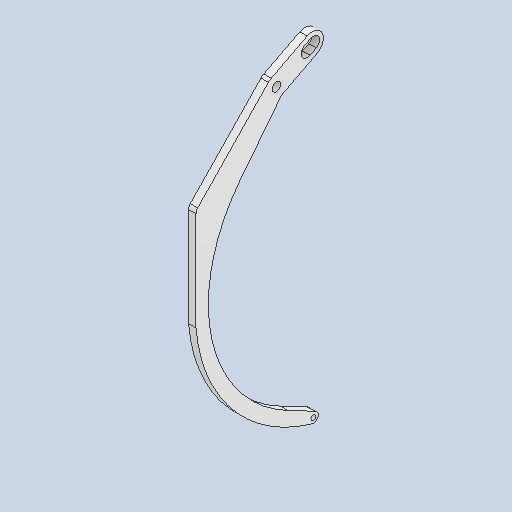
# Autodesk Inventor part: hand-grab-v1-MDF-arm
Saved by Autodesk Inventor 2025.2 (Build 292293000, 293)
## iProperties
Created: 2024-10-30
Part Number: hand-grab-v1-MDF-arm
Material: ABS プラスチック
Document SubType Name: Modeling
Designer: haruy
Density: 1.06 g/cm^3
Appearance: 滑らか - 白
Author: haruy
Autodesk Inventor part; units mm, degrees
ref_plane "YZ Plane" through (0, 0, 0) normal (1, 0, 0) x (0, 1, 0)
ref_plane "XZ Plane" through (0, 0, 0) normal (0, 1, 0) x (-1, 0, 0)
ref_plane "XY Plane" through (0, 0, 0) normal (0, 0, 1) x (1, 0, 0)
derived "hand-grab-v3-Sketch-Base.ipt"
sketch "スケッチ1" plane through (400, 0, 0) normal (1, 0, 0) x (0, 1, 0)
  circle A0 centre (0, 0) radius 120 construction
  circle A1 centre (-96.5237, 35.1318) radius 6.5
  line L0 (0, 0) -> (-96.5237, 35.1318)
  line L1 (0, 0) -> (0, 120)
  line L2 (246.0862, 200) -> (-251.4603, 200)
  circle A2 centre (-67.6203, 200) radius 6.5
  line L3 (0, 0) -> (-120, 0)
  line L4 (248, 9.15) -> (186, 9.15)
  line L5 (186, 9.15) -> (186, -9.15)
  line L6 (186, -9.15) -> (248, -9.15)
  line L7 (248, -9.15) -> (248, 9.15)
  line L8 (186, 5.15) -> (178, 5.15)
  line L9 (178, 5.15) -> (178, -4.85)
  line L10 (178, -4.85) -> (186, -4.85)
  line L11 (186, -4.85) -> (186, 5.15)
  line L12 (178, 3.15) -> (173, 3.15)
  line L13 (173, 3.15) -> (173, -2.85)
  line L14 (173, -2.85) -> (178, -2.85)
  line L15 (178, -2.85) -> (178, 3.15)
  line L16 (173, 2.65) -> (158, 2.65)
  line L17 (158, 2.65) -> (158, -2.35)
  line L18 (158, -2.35) -> (173, -2.35)
  line L19 (173, -2.35) -> (173, 2.65)
  line L20 (186, 34.15) -> (184, 34.15)
  line L21 (184, 34.15) -> (184, -47.85)
  line L22 (184, -47.85) -> (186, -47.85)
  line L23 (186, -47.85) -> (186, 34.15)
  circle A3 centre (150, 65) radius 4 construction
  circle A4 centre (150, 65) radius 14 construction
  line L24 (186, 34.15) -> (191, 34.15)
  line L25 (191, 34.15) -> (191, 14.15)
  line L26 (191, 14.15) -> (186, 14.15)
  line L27 (186, 14.15) -> (186, 34.15)
  line L28 (184, 34.15) -> (147.5804, 61.8148) construction
  line L29 (151.3835, 68.7531) -> (191, 54.15) construction
  line L30 (191, 54.15) -> (191, 34.15)
  line L31 (239.3868, 130) -> (-239.3868, 130)
  circle A5 centre (-96.5237, 35.1318) radius 4
  circle A6 centre (150, 65) radius 9
  line L32 (-92.7649, 33.7637) -> (-100.2825, 36.4998)
  line L33 (165, 36) -> (150, 36) construction
  circle A7 centre (150, 36) radius 5 construction
  circle A8 centre (150, 36) radius 9 construction
  circle A9 centre (-98.8174, 128.095) radius 6.5
  circle A10 centre (165, 36) radius 5 construction
  line L34 (150, 65) -> (165, 36) construction
  circle A11 centre (165, 36) radius 9
  circle A12 centre (150, 65) radius 41.6497 construction
  line L35 (150, 65) -> (150, 36) construction
  line L36 (150, 65) -> (-96.5237, 35.1318) construction
  line L37 (-98.8174, 128.095) -> (150, 65) construction
  line L38 (150, 65) -> (150, 23.3503)
  circle A13 centre (150, 65) radius 32.6497 construction
  circle A14 centre (150, 32.3503) radius 9 construction
  line L39 (166.9362, 23.3503) -> (134.8586, 23.3503)
  line L40 (174, 3.15) -> (174, -2.85)
  circle A15 centre (-96.5237, 35.1318) radius 2
  circle A16 centre (150, 65) radius 3.5
  circle A17 centre (150, 65) radius 29 construction
  circle A18 centre (163.3233, 39.2417) radius 5 construction
  circle A19 centre (162.8638, 40.1299) radius 5
  line L41 (150, 65) -> (169.1348, 28.006) construction
  circle A20 centre (165.4594, 35.1118) radius 5
  line L42 (167.3049, 42.427) -> (169.9005, 37.4089)
  line L43 (158.4228, 37.8328) -> (161.0183, 32.8147)
  circle A21 centre (25, 0) radius 120
  circle A22 centre (25, 0) radius 122.5
  circle A23 centre (25, 0) radius 130.5
  line L44 (-92.7649, 33.7637) -> (-81.3303, 55.6226)
  line L45 (25, 130.5) -> (95, 130.5)
  line L46 (95, 130.5) -> (156.2451, 71.4806)
  line L47 (157.994, 69.1348) -> (172.994, 40.1348)
  line L48 (157.006, 31.8652) -> (142.006, 60.8652)
  line L49 (142.006, 60.8652) -> (98.8819, 94.5593)
  circle A24 centre (123.9097, 89.024) radius 1.5
  circle A25 centre (25, 125.5) radius 1.5
  circle A26 centre (-61, 92) radius 1.5
  line L50 (170, -52.2973) -> (211.3465, -67.3462)
  line L51 (211.3465, -67.3462) -> (205.1901, -84.2607)
  line L52 (205.1901, -84.2607) -> (163.8436, -69.2118)
  line L53 (163.8436, -69.2118) -> (170, -52.2973)
  line L54 (166.9218, -60.7546) -> (0, 0)
  line L55 (172.8191, -53.3234) -> (166.6627, -70.2379)
  line L56 (186, -47.85) -> (172.8191, -53.3234)
  line L57 (182.216, -56.7436) -> (176.0596, -73.6581)
  line L58 (186, -47.85) -> (191, -47.85)
  line L59 (191, -47.85) -> (191, -37.85)
  line L60 (191, -37.85) -> (186, -37.85)
  line L61 (186, -37.85) -> (186, -47.85)
  line L62 (191, -47.85) -> (182.216, -56.7436)
  circle A27 centre (221.5, -275) radius 6
  line L63 (211.5, 20) -> (208.5, 20)
  line L64 (208.5, 20) -> (208.5, -53.7075)
  line L65 (208.5, -53.7075) -> (211.5, -53.7075)
  line L66 (211.5, -53.7075) -> (211.5, 20)
  line L67 (211.5, 20) -> (231.5, 20)
  line L68 (231.5, 20) -> (231.5, -53.7075)
  line L69 (231.5, -53.7075) -> (211.5, -53.7075)
  line L70 (211.5, -53.7075) -> (211.5, 20)
  line L71 (-432.3334, -230) -> (-447.3334, -230)
  line L72 (-447.3334, -230) -> (-447.3334, -860)
  line L73 (-447.3334, -860) -> (-432.3334, -860)
  line L74 (-432.3334, -860) -> (-432.3334, -230)
  line L75 (-432.3334, -250) -> (-432.3334, -230)
  line L76 (343, -291.5) -> (278.5, -291.5)
  line L77 (278.5, -291.5) -> (278.5, -334.5)
  line L78 (278.5, -334.5) -> (343, -334.5)
  line L79 (343, -334.5) -> (343, -291.5)
  line L80 (278.5, -291.5) -> (293.5, -291.5)
  line L81 (293.5, -291.5) -> (293.5, -276.5)
  line L82 (293.5, -276.5) -> (278.5, -276.5)
  line L83 (278.5, -276.5) -> (278.5, -291.5)
  line L84 (211.5, -53.7075) -> (231.5, -53.7075)
  line L85 (231.5, -53.7075) -> (231.5, -305) construction
  line L86 (231.5, -305) -> (211.5, -305)
  line L87 (211.5, -305) -> (211.5, -53.7075) construction
  line L88 (-432.3334, -303) -> (-447.3334, -303)
  line L89 (-432.3334, -303) -> (875.6666, -303)
  line L90 (875.6666, -303) -> (875.6666, -323)
  line L91 (875.6666, -323) -> (-432.3334, -323)
  line L92 (-432.3334, -323) -> (-432.3334, -303)
  line L93 (278.5, -334.5) -> (293.5, -334.5)
  line L94 (293.5, -334.5) -> (293.5, -349.5)
  line L95 (293.5, -349.5) -> (278.5, -349.5)
  line L96 (278.5, -349.5) -> (278.5, -334.5)
  line L97 (278.5, -276.5) -> (263.5, -276.5)
  line L98 (263.5, -276.5) -> (263.5, -359.5)
  line L99 (263.5, -359.5) -> (278.5, -359.5)
  line L100 (278.5, -359.5) -> (278.5, -276.5)
  circle A28 centre (221.5, -275) radius 15
  line L101 (231.5, -275) -> (211.5, -275)
  line L102 (211.5, -275) -> (211.5, -305)
  line L103 (211.5, -305) -> (231.5, -305)
  line L104 (231.5, -305) -> (231.5, -275)
  line L105 (226.5, -266.3397) -> (216.5, -283.6603)
  line L106 (242.4808, -298.6603) -> (252.4808, -281.3397)
  line L107 (216.5, -283.6603) -> (242.4808, -298.6603)
  line L108 (-524.3334, 10.1879) -> (-524.3334, -1075.6286)
  line L109 (278.5, -349.5) -> (263.5, -349.5)
  line L110 (278.5, -276.5) -> (225.8253, -260.6372)
  line L111 (263.5, -349.5) -> (209.9279, -284.544)
  line L112 (278.5, -313) -> (263.5, -313)
  circle A29 centre (271, -291.5) radius 1.6
  circle A30 centre (271, -334.5) radius 1.6
  circle A31 centre (221.5, -275) radius 9.1
  circle A32 centre (221.5, -275) radius 50
  circle A33 centre (239.5, -334.8519) radius 12.5
  line L113 (221.5, -275) -> (237.3114, -322.4342)
  line L114 (221.5, -275) -> (178.1987, -300)
  line L115 (221.5, -275) -> (221.5, -225)
  line L116 (221.5, -275) -> (254.6735, -237.5899)
  circle A34 centre (259.5, -334.8519) radius 4
  circle A35 centre (239.5, -354.8519) radius 4
  circle A36 centre (219.5, -334.8519) radius 4
  line L117 (206.6714, -277.2613) -> (215.5457, -335.4549)
  line L118 (216.6716, -337.6803) -> (236.6716, -357.6803)
  line L119 (263.5, -349.5) -> (240.9941, -358.5624)
  circle A37 centre (259.5, -334.8519) radius 1.6
  circle A38 centre (239.5, -354.8519) radius 1.6
  circle A39 centre (219.5, -334.8519) radius 1.6
  point P0 (-60, 0)
  point P1 (95.5189, 130)
  point P2 (13.5873, 130)
  point P3 (-100.3663, 36.2426)
  point P4 (-92.6811, 34.0209)
  point P5 (-92.7432, 33.8053)
  point P6 (875.6666, -313)
  point P7 (186, 0.15)
  point P8 (186, 0)
  dimension "d1" = 4
  dimension "d2" = 7
  dimension "d3" = 10
  dimension "d4" = 10
  dimension "d5" = 1
  dimension "d6" = 10
  dimension "d7" = 1
  dimension "d8" = 70
  dimension "d12" = 3
  dimension "d13" = 3
  dimension "d14" = 3
  dimension "d15" = 5
  dimension "d16" = 0
  dimension "d17" = 61
  dimension "d18" = 92
  dimension "d19" = 98.9097
  dimension "d20" = 89.024
  measures "d1" diameter of A15
  measures "d2" diameter of A16
  measures "d3" diameter of A18
  measures "d4" diameter of A19
  measures "d5" distance of A19.centre A18.centre
  measures "d6" diameter of A20
  measures "d7" distance of L33.start A20.centre
  measures "d8" horizontal distance of A22.centre L45.end
  measures "d12" diameter of A24
  measures "d13" diameter of A25
  measures "d14" diameter of A26
  measures "d15" distance from line of A25.centre L45
  measures "d16" horizontal distance of A25.centre L45.start
  measures "d17" horizontal distance of A26.centre point (0, 0)
  measures "d18" distance from line of L3 A26.centre
  measures "d19" horizontal distance of A24.centre A22.centre
  measures "d20" vertical distance of A22.centre A24.centre
sketch "スケッチ2" plane through (0, 400, 0) normal (0, 1, 0) x (-1, 0, 0)
  circle A0 centre (0, 0) radius 120
  line L0 (0, 0) -> (-331.4625, 0)
  line L1 (67.5, -116.9134) -> (-135, 0)
  circle A1 centre (0, 0) radius 5
  line L2 (0, 0) -> (67.5, 116.9134)
  line L3 (0, 0) -> (67.5, -116.9134)
  line L4 (0, 0) -> (-135, 0)
  line L5 (17.0359, 37.507) -> (12.0359, 28.8468)
  line L6 (12.0359, 28.8468) -> (15.5, 26.8468)
  line L7 (15.5, 26.8468) -> (20.5, 35.507)
  line L8 (20.5, 35.507) -> (17.0359, 37.507)
  line L9 (20.5, 35.507) -> (15.5, 26.8468)
  line L10 (15.5, 26.8468) -> (18.9641, 24.8468)
  line L11 (18.9641, 24.8468) -> (23.9641, 33.507)
  line L12 (23.9641, 33.507) -> (20.5, 35.507)
  line L13 (14.5359, 33.1769) -> (21.4641, 29.1769)
  circle A2 centre (0, 0) radius 2.65
  line L14 (16.8194, 37.632) -> (10.3194, 26.3737)
  line L15 (10.3194, 26.3737) -> (5.9893, 28.8737)
  line L16 (5.9893, 28.8737) -> (12.4893, 40.132)
  line L17 (12.4893, 40.132) -> (16.8194, 37.632)
  line L18 (28.5107, 30.882) -> (24.1806, 33.382)
  line L19 (22.0107, 19.6237) -> (28.5107, 30.882)
  line L20 (24.1806, 33.382) -> (17.6806, 22.1237)
  line L21 (17.6806, 22.1237) -> (22.0107, 19.6237)
  circle A3 centre (0, 0) radius 28.3207
  line L22 (-41, 9.25) -> (-41, 4.25)
  line L23 (-41, 4.25) -> (-28, 4.25)
  line L24 (-28, 9.25) -> (-41, 9.25)
  line L25 (-28, 4.25) -> (-28, 9.25)
  line L26 (-41, -4.25) -> (-28, -4.25)
  line L27 (-41, -9.25) -> (-41, -4.25)
  line L28 (-28, -9.25) -> (-41, -9.25)
  line L29 (-28, -4.25) -> (-28, -9.25)
  line L30 (12.4893, -40.132) -> (16.8194, -37.632)
  line L31 (16.8194, -37.632) -> (10.3194, -26.3737)
  line L32 (5.9893, -28.8737) -> (12.4893, -40.132)
  line L33 (10.3194, -26.3737) -> (5.9893, -28.8737)
  line L34 (24.1806, -33.382) -> (17.6806, -22.1237)
  line L35 (28.5107, -30.882) -> (24.1806, -33.382)
  line L36 (22.0107, -19.6237) -> (28.5107, -30.882)
  line L37 (17.6806, -22.1237) -> (22.0107, -19.6237)
  line L38 (5.9893, 28.8737) -> (5.373, 27.8064)
  line L39 (22.0107, 19.6237) -> (21.3945, 18.5564)
  line L40 (-28, 9.25) -> (-26.7675, 9.25)
  line L41 (-28, -9.25) -> (-26.7675, -9.25)
  line L42 (5.9893, -28.8737) -> (2.1934, -22.2991)
  line L43 (22.0107, -19.6237) -> (21.3945, -18.5564)
  line L44 (13.6109, 31.5748) -> (3.6109, 14.2543)
  line L45 (3.6109, 14.2543) -> (-1.5853, 17.2543)
  line L46 (-1.5853, 17.2543) -> (8.4147, 34.5748)
  line L47 (8.4147, 34.5748) -> (13.6109, 31.5748)
  circle A4 centre (3.5128, 20.0844) radius 1.5
  circle A5 centre (8.5128, 28.7446) radius 1.5
  circle A6 centre (20.6372, 21.7446) radius 1.5
  circle A7 centre (15.6372, 13.0844) radius 1.5
  circle A8 centre (-29.15, 7) radius 1.5
  circle A9 centre (-19.15, 7) radius 1.5
  circle A10 centre (-19.15, -7) radius 1.5
  circle A11 centre (-29.15, -7) radius 1.5
  circle A12 centre (8.5128, -28.7446) radius 1.5
  circle A13 centre (3.5128, -20.0844) radius 1.5
  circle A14 centre (15.6372, -13.0844) radius 1.5
  circle A15 centre (20.6372, -21.7446) radius 1.5
  line L48 (1.0128, 15.7543) -> (13.6109, 31.5748)
  circle A16 centre (0, 0) radius 34.3835
  line L49 (-8, 47) -> (-188, 47)
  line L50 (-188, 47) -> (-188, 32)
  line L51 (-188, 32) -> (-8, 32)
  line L52 (-8, 32) -> (-8, 47)
ref_plane "作業平面1" through (400, 0, 0) normal (1, 0, 0) x (0, 1, 0)
ref_plane "作業平面2" through (0, 400, 0) normal (0, 1, 0) x (-1, 0, 0)
extrude "押し出し1" add sketch "スケッチ1" against normal blind 6 contours L44 A22 A1 | A1 A22 L1 A21 L44 | A22 A5 A23 A1 | A1 A23 L31 L49 A22 | A22 L49 A21 L1 | A5 L0 A15 L32 | A5 L32 A15 L0 | L31 L46 A6 L49 A23 | A6 | A6 L38 L48 | L38 A6 L47 A11 A19 L48 | A11 A19 L43 A20 L42 | A24 | A25 | A26
fillet "フィレット1" radius 5 1 edges at (397, 95.5189, 130)
sketch "スケッチ3" plane through (400, 13.5873, 130) normal (1, 0, 0) x (0, 0, -1)
  circle A0 centre (65, 136.4127) radius 3.5 projected
  arc A1 (87.573, 153.7176) -> (92.1672, 144.8355) centre (89.8701, 149.2766) ccw projected
  line L0 (87.573, 153.7176) -> (92.5911, 156.3132) projected
  arc A2 (97.1853, 147.431) -> (92.5911, 156.3132) centre (94.8882, 151.8721) ccw projected
  line L1 (97.1853, 147.431) -> (92.1672, 144.8355) projected
  circle A3 centre (94.8682, -110.111) radius 2 projected
  arc A4 (1.3997, 83.384) -> (0, 79.9145) centre (5, 79.9145) ccw projected
  line L2 (0, 79.9145) -> (0, 0) projected
  arc A5 (0, 0) -> (93.7574, -113.9536) centre (130, 11.4127) ccw projected
  arc A6 (93.7574, -113.9536) -> (95.9791, -106.2683) centre (94.8682, -110.111) ccw projected
  arc A7 (95.9791, -106.2683) -> (96.1947, -106.3305) centre (130, 11.4127) ccw projected
  line L3 (96.1947, -106.3305) -> (74.3774, -94.9176) projected
  arc A8 (35.4407, 85.2946) -> (74.3774, -94.9176) centre (130, 11.4127) ccw projected
  line L4 (35.4407, 85.2946) -> (69.1348, 128.4188) projected
  line L5 (69.1348, 128.4188) -> (98.1348, 143.4188) projected
  arc A9 (98.1348, 143.4188) -> (89.8652, 159.4067) centre (94, 151.4127) ccw projected
  line L6 (89.8652, 159.4067) -> (60.8652, 144.4067) projected
  arc A10 (60.8652, 144.4067) -> (58.5194, 142.6578) centre (65, 136.4127) ccw projected
  line L7 (58.5194, 142.6578) -> (1.3997, 83.384) projected
  point P0 (130, -13.5873)
